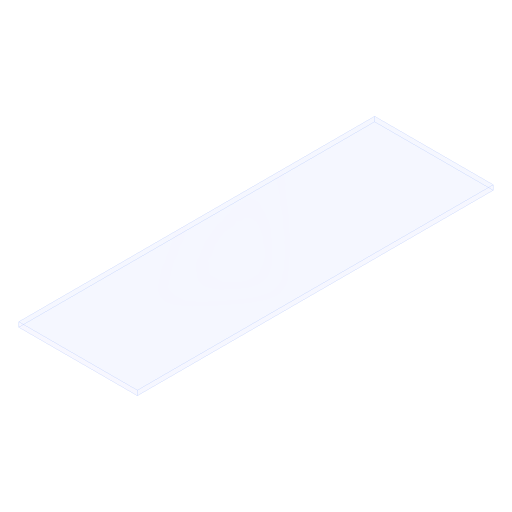
# Autodesk Inventor part: Microscope slide
Saved by Autodesk Inventor 2023 (Build 270158000, 158)
## iProperties
Created: 2022-09-28
Part Number: Microscope slide
Material: Generic
Document SubType Name: Modeling
Designer: ferrerx
Density: 1 g/cm^3
Appearance: Clear - Blue
Author: ferrerx
Autodesk Inventor part; units mm, degrees
ref_plane "YZ Plane" through (0, 0, 0) normal (1, 0, 0) x (0, 1, 0)
ref_plane "XZ Plane" through (0, 0, 0) normal (0, 1, 0) x (-1, 0, 0)
ref_plane "XY Plane" through (0, 0, 0) normal (0, 0, 1) x (1, 0, 0)
sketch "Sketch1" plane through (0, 0, 0) normal (0, 1, 0) x (-1, 0, 0)
  line L0 (-12.5, 37.5) -> (12.5, 37.5)
  line L1 (12.5, 37.5) -> (12.5, -37.5)
  line L2 (12.5, -37.5) -> (-12.5, -37.5)
  line L3 (-12.5, -37.5) -> (-12.5, 37.5)
  line L4 (-12.5, 37.5) -> (12.5, -37.5) construction
  line L5 (12.5, 37.5) -> (-12.5, -37.5) construction
  point P0 (0, 0)
  dimension "d0" = 75
  dimension "d1" = 25
  constraints: 12 end point, 2 midpoint, 2 parallel, 1 horizontal, 1 perpendicular
  measures "d0" distance of L0.end L1.end
  measures "d1" distance of L1.end L2.end
extrude "Extrusion1" add sketch "Sketch1" along normal blind 1
body "Solid1"
